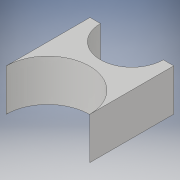
# Autodesk Inventor part: Part26
Saved by Autodesk Inventor 2019 (Build 230136000, 136)
## iProperties
Created: 2021-08-31
Part Number: Part26
Material: 一般
Document SubType Name: Sheet Metal
Designer: yuta
Density: 1 g/cm^3
Sheet Metal Rule: Default_mm
Appearance: 既定
Author: yuta
Autodesk Inventor part; units mm, degrees
ref_plane "YZ Plane" through (0, 0, 0) normal (1, 0, 0) x (0, 1, 0)
ref_plane "XZ Plane" through (0, 0, 0) normal (0, 1, 0) x (-1, 0, 0)
ref_plane "XY Plane" through (0, 0, 0) normal (0, 0, 1) x (1, 0, 0)
sketch "スケッチ1" plane through (0, 0, 0) normal (0, 1, 0) x (-1, 0, 0)
  line L0 (4.6641, 14.0328) -> (-35.3359, 14.0328)
  line L1 (-35.3359, 14.0328) -> (-35.3359, -25.9672)
  line L2 (-35.3359, -25.9672) -> (4.6641, -25.9672)
  line L3 (4.6641, -25.9672) -> (4.6641, 14.0328)
  point P0 (0, 0)
  dimension "d0" = 40
  dimension "d1" = 40
  constraints: 8 end point, 2 parallel, 1 horizontal, 1 perpendicular
  measures "d0" distance of L2.end L1.end
  measures "d1" distance of L1.end L0.end
extrude "押し出し1" add sketch "スケッチ1" along normal blind 20
sketch "スケッチ2" plane through (0, 20, 0) normal (0, 1, 0) x (1, 0, 0)
  line L0 (35.3359, 25.9672) -> (-4.6641, 25.9672) projected
  circle A0 centre (15.3359, 25.9672) radius 15
  line L1 (-4.6641, -14.0328) -> (35.3359, -14.0328) projected
  circle A1 centre (15.3359, -14.2518) radius 20.0012
  point P0 (0, 0)
  dimension "d4" = 30
  constraints: 1 centre point, 1 midpoint, 3 other
  measures "d4" diameter of A0
hole "穴1" at (15.3359, 20, 14.2518) direction (0, -1, 0) diameter 40 depth 20
sketch "スケッチ3" plane through (0, 20, 0) normal (0, 1, 0) x (1, 0, 0)
  line L0 (35.3359, 25.9672) -> (-4.6641, 25.9672) projected
  circle A0 centre (15.3359, 25.9672) radius 15
  point P0 (0, 0)
  dimension "d12" = 30
  constraints: 1 centre point, 1 midpoint
  measures "d12" diameter of A0
hole "穴2" at (15.3359, 20, -25.9672) direction (0, -1, 0) diameter 30 depth 20
equation "\"BendRadius\" = Thickness"
equation "\"BendReliefWidth\" = Thickness"
equation "\"BendReliefDepth\" = 0.5 * Thickness"
equation "\"CornerReliefSize\" = 4 * Thickness"
equation "\"MinimumRemnant\" = 2 * Thickness"
equation "\"TransitionRadius\" = BendRadius"
equation "\"JacobiRadiusSize\" = BendRadius"
equation "\"GapSize\" = Thickness"
equation "\"Thickness\" = 0.5"
